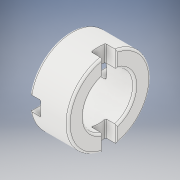
# Autodesk Inventor part: MOR-20C  Sleeve
Saved by Autodesk Inventor 2019 (Build 230136000, 136)
## iProperties
Created: 2024-03-13
Part Number: MOR-20C  Sleeve
Material: Generic
Catalog Web Link: www.cadenas.de
Description: MOR-C Sleeve-
Vendor: NBK
Document SubType Name: Modeling
Designer: psAdmin
Manufacturer: NBK
Mass: 1.6963 g
Surface Area: 13.1042 cm^2
Volume: 1.6963 cm^3
Density: 1 g/cm^3
Appearance: PSOLRGB-255-255-255
Category: PARTsolutions
Company: NBK
Title: MOR-20C  Sleeve
Author: Cadenas PARTsolutions
PSOL_IDENT_0: {$CADENAS_DATA/23d-libs/nbk/motion_control_parts/couplicon_mini/oldham_type/mor/mor_c_2.prj},177 {VT
PSOL_IDENT_1: YP=3D},{NB=MOR-20C  Sleeve},{LINA=MOR-20C  Sleeve},{NN=MOR-C Sleeve},{DATE=12.03.2024 08:53:06},{GEO
PSOL_IDENT_2: MDATE=21.12.2021 07:27:30},{VERSION=},{LINEID=720},{WBVAR=},{WBNUMERIC=}  {NB=MOR-20C  Sleeve},{LINA=
PSOL_IDENT_3: MOR-20C  Sleeve},{KT=DUMMY},{CN=MOR-20C},{A=20},{L=8.75},{W=27.4},{E=12.2},{F=4.38},{G=7.5},{M=M2.5}
PSOL_IDENT_4: ,{RZ=0.25},{KV=2.70},{KD=3.50},{KK=0.3},{SR=0.50}
NB: MOR-20C  Sleeve
NN: MOR-C Sleeve
NBSYN: $CN.  Sleeve
LINA: MOR-20C  Sleeve
CATALOG: NBK (Nabeya Bi-tech Kaisha
CN: MOR-20C
A: 20
L: 8.75
W: 27.4
E: 12.2
F: 4.38
G: 7.5
M: M2.5
RZ: 0.25
KV: 2.7
KD: 3.5
KK: 0.3
SR: 0.5
SUPPLIER: NBK
ARTICLENO: MOR-20C  Sleeve
BOMINFO: MOR-20C  Sleeve
CREATOR: CADENAS GmbH
Autodesk Inventor part; units mm, degrees
sketch "Sketch_1" plane through (0, 0, 0) normal (0, 0, 1) x (1, 0, 0)
  line L0 (9.4, 0) -> (0, 0)
  arc A0 (0, 6.6) -> (0.5, 6.1) centre (0.5, 6.6) ccw
  line L1 (0.5, 6.1) -> (8.9, 6.1)
  arc A1 (8.9, 6.1) -> (9.4, 6.6) centre (8.9, 6.6) ccw
  line L2 (9.4, 6.6) -> (9.4, 9.5)
  arc A2 (9.4, 9.5) -> (8.9, 10) centre (8.9, 9.5) ccw
  line L3 (8.9, 10) -> (0.5, 10)
  arc A3 (0.5, 10) -> (0, 9.5) centre (0.5, 9.5) ccw
  line L4 (0, 9.5) -> (0, 6.6)
  constraints: 10 end point, 8 point on circle, 4 centre point
revolve "Revolution1" add sketch "Sketch_1" angle 360 about axis through (9.4, 0, 0) along (1, 0, 0)
sketch "Sketch_2" plane through (0, 0, 0) normal (0, 0, 1) x (1, 0, 0)
  line L0 (-1, -2) -> (0, -2)
  arc A0 (0.25, -1.75) -> (0, -2) centre (0.25, -2) ccw
  line L1 (0.25, -1.75) -> (2.4, -1.75)
  arc A1 (2.4, -1.75) -> (2.7, -1.45) centre (2.4, -1.45) ccw
  line L2 (2.7, -1.45) -> (2.7, 1.45)
  arc A2 (2.7, 1.45) -> (2.4, 1.75) centre (2.4, 1.45) ccw
  line L3 (2.4, 1.75) -> (0.25, 1.75)
  arc A3 (0, 2) -> (0.25, 1.75) centre (0.25, 2) ccw
  line L4 (0, 2) -> (-1, 2)
  line L5 (-1, 2) -> (-1, -2)
  constraints: 12 end point, 8 point on circle, 4 centre point
extrude "Extrusion1" cut sketch "Sketch_2" along normal mid plane 20
sketch "Sketch_3" plane through (0, 0, 0) normal (0, 1, 0) x (-1, 0, 0)
  arc A0 (-6.7, 1.45) -> (-7, 1.75) centre (-7, 1.45) ccw
  line L0 (-7, 1.75) -> (-9.15, 1.75)
  arc A1 (-9.4, 2) -> (-9.15, 1.75) centre (-9.15, 2) ccw
  line L1 (-9.4, 2) -> (-10.4, 2)
  line L2 (-10.4, 2) -> (-10.4, -2)
  line L3 (-10.4, -2) -> (-9.4, -2)
  arc A2 (-9.15, -1.75) -> (-9.4, -2) centre (-9.15, -2) ccw
  line L4 (-9.15, -1.75) -> (-7, -1.75)
  arc A3 (-7, -1.75) -> (-6.7, -1.45) centre (-7, -1.45) ccw
  line L5 (-6.7, -1.45) -> (-6.7, 1.45)
  constraints: 12 end point, 8 point on circle, 4 centre point
extrude "Extrusion2" cut sketch "Sketch_3" along normal mid plane 20
ref_plane "p2_p1_XY" through (0, 0, 0) normal (1, 0, 0) x (0, 0, -1)
ref_plane "p2_p1_YZ" through (0, 0, 0) normal (0, 0, -1) x (0, 1, 0)
ref_plane "p2_p1_ZX" through (0, 0, 0) normal (0, 1, 0) x (1, 0, 0)
ref_plane "p2_p3_XY" through (9.4, 0, 0) normal (-1, 0, 0) x (0, 0, -1)
ref_plane "p2_p3_YZ" through (9.4, 0, 0) normal (0, 0, -1) x (0, -1, 0)
ref_plane "p2_p3_ZX" through (9.4, 0, 0) normal (0, -1, 0) x (-1, 0, 0)
body "Solid1"
